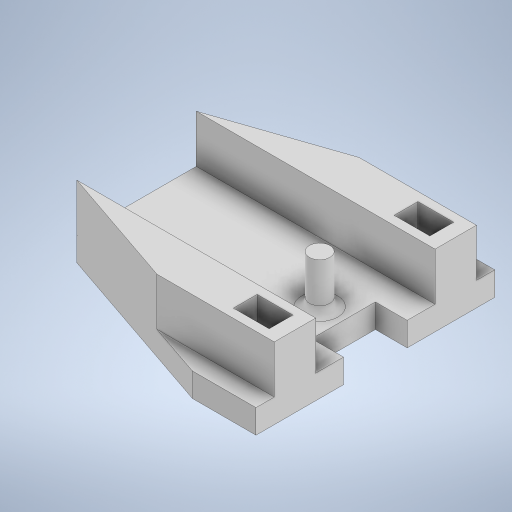
# Autodesk Inventor part: IRMount
Saved by Autodesk Inventor 2024.2 (Build 282272000, 272)
## iProperties
Created: 2024-04-04
Part Number: IRMount
Material: Generic
Document SubType Name: Modeling
Designer: ringl
Density: 1 g/cm^3
Appearance: Default
Author: ringl
Autodesk Inventor part; units mm, degrees
ref_plane "YZ Plane" through (0, 0, 0) normal (1, 0, 0) x (0, 1, 0)
ref_plane "XZ Plane" through (0, 0, 0) normal (0, 1, 0) x (-1, 0, 0)
ref_plane "XY Plane" through (0, 0, 0) normal (0, 0, 1) x (1, 0, 0)
sketch "Sketch1" plane through (0, 0, 0) normal (0, 1, 0) x (-1, 0, 0)
  line L0 (0, 0) -> (8, 0)
  line L1 (8, -30) -> (0, -30)
  line L2 (0, -30) -> (0, 0)
  line L3 (6.25, -3.4) -> (1.75, -3.4)
  line L4 (1.75, -3.4) -> (1.75, -6.4)
  line L5 (1.75, -6.4) -> (6.25, -6.4)
  line L6 (6.25, -6.4) -> (6.25, -3.4)
  line L7 (6.25, -23.6) -> (1.75, -23.6)
  line L8 (1.75, -23.6) -> (1.75, -26.6)
  line L9 (1.75, -26.6) -> (6.25, -26.6)
  line L10 (6.25, -26.6) -> (6.25, -23.6)
  line L11 (8, 0) -> (30, -7.5)
  line L12 (30, -7.5) -> (30, -22.5)
  line L13 (30, -22.5) -> (8, -30)
  dimension "d0" = 30
  dimension "d1" = 8
  dimension "d2" = 4.5
  dimension "d3" = 3
  dimension "d4" = 3
  dimension "d5" = 17.2
  dimension "d6" = 3.4
  dimension "d7" = 1.75
  dimension "d8" = 15
  dimension "d10" = 7.5
  dimension "d11" = 22
  dimension "d12" = 22
  constraints: 28 end point, 5 parallel, 3 horizontal, 2 perpendicular, 2 point on line, 1 vertical
  measures "d0" distance between parallel lines of L0 L1
  measures "d1" distance of L1.start L1.end
  measures "d2" distance of L4.end L5.end
  measures "d3" distance of L3.end L4.end
  measures "d4" distance of L7.end L8.end
  measures "d5" distance between parallel lines of L7 L5
  measures "d6" distance between parallel lines of L0 L3
  measures "d7" distance between parallel lines of L2 L8
  measures "d8" distance of L11.end L12.end
  measures "d10" vertical distance of L0.end L11.end
  measures "d11" distance from line of L1.start L12
  measures "d12" horizontal distance of L0.end L11.end
extrude "Extrusion1" add sketch "Sketch1" along normal blind 3
sketch "Sketch2" plane through (0, 3, 0) normal (0, 1, 0) x (1, 0, 0)
  circle A0 centre (-7, 15) radius 1.3
  line L0 (-30, 22.5) -> (-30, 7.5) projected
  line L1 (-30, 7.5) -> (0, 7.5)
  line L2 (-30, 22.5) -> (0, 22.5)
  line L3 (-30, 7.5) -> (-14.7467, 2.3)
  line L4 (-30, 7.5) -> (-8, 0) projected
  line L5 (0, 0) -> (0, 30) projected
  line L6 (0, 2.3) -> (0, 7.5)
  line L7 (0, 2.3) -> (-14.7467, 2.3)
  line L8 (-8, 30) -> (-30, 22.5) projected
  line L9 (-30, 22.5) -> (-14.7467, 27.7)
  line L10 (-14.7467, 27.7) -> (0, 27.7)
  line L11 (0, 27.7) -> (0, 22.5)
  line L12 (-8, 0) -> (0, 0) projected
  line L13 (-1.75, 3.4) -> (-6.25, 3.4) projected
  line L14 (-6.25, 26.6) -> (-1.75, 26.6) projected
  point P0 (0, 27.7)
  dimension "d17" = 2.6
  dimension "d21" = 1.1
  dimension "d22" = 1.1
  dimension "d23" = 15
  dimension "d24" = 7
  constraints: 16 end point, 4 point on line, 2 horizontal, 2 perpendicular, 1 centre point, 1 collinear, 1 parallel
  measures "d17" diameter of A0
  measures "d21" distance between parallel lines of L13 L7
  measures "d22" distance between parallel lines of L10 L14
  measures "d23" distance from line of L12 A0.centre
  measures "d24" distance from line of L5 A0.centre
extrude "Extrusion2" add sketch "Sketch2" along normal blind 6 contours A0 | L8 L10 L5 L2 | L1 L5 L7 L3
sketch "Sketch3" plane through (0, 0, 0) normal (0, -1, 0) x (1, 0, 0)
  line L0 (-1.75, -6.4) -> (-1.75, -3.4) projected
  line L1 (-1.75, -3.4) -> (-6.25, -3.4)
  line L2 (-6.25, -3.4) -> (-6.25, -6.4)
  line L3 (-6.25, -6.4) -> (-1.75, -6.4)
  line L4 (-1.75, -6.4) -> (-1.75, -3.4)
  line L5 (-1.75, -26.6) -> (-1.75, -23.6) projected
  line L6 (-6.25, -26.6) -> (-1.75, -26.6) projected
  line L7 (-1.75, -23.6) -> (-6.25, -23.6)
  line L8 (-6.25, -23.6) -> (-6.25, -26.6)
  line L9 (-6.25, -26.6) -> (-1.75, -26.6)
  line L10 (-1.75, -26.6) -> (-1.75, -23.6)
  point P0 (0, 0)
  constraints: 16 end point, 4 parallel, 2 horizontal, 2 perpendicular
extrude "Extrusion3" cut sketch "Sketch3" against normal through all
sketch "Sketch4" plane through (0, 3, 0) normal (0, 1, 0) x (1, 0, 0)
  line L0 (0, 7.5) -> (0, 22.5) projected
  line L1 (0, 11) -> (-4, 11)
  line L2 (-4, 11) -> (-4, 19)
  line L3 (-4, 19) -> (0, 19)
  line L4 (0, 19) -> (0, 11)
  circle A0 centre (-7, 15) radius 1.3 projected
  line L5 (0, 7.5) -> (-30, 7.5) projected
  point P0 (0, 0)
  point P1 (0, 19)
  dimension "d29" = 3
  dimension "d30" = 8
  dimension "d31" = 3.5
  constraints: 8 end point, 2 parallel, 1 horizontal, 1 perpendicular, 1 point on line
  measures "d29" distance from line of A0.centre L2
  measures "d30" distance of L1.end L2.end
  measures "d31" distance between parallel lines of L1 L5
extrude "Extrusion4" cut sketch "Sketch4" against normal through all contours L1 L2 L3 L0
fillet "Fillet1" radius 1 1 edges at (-8.3, 3, -15)
body "Solid1"
